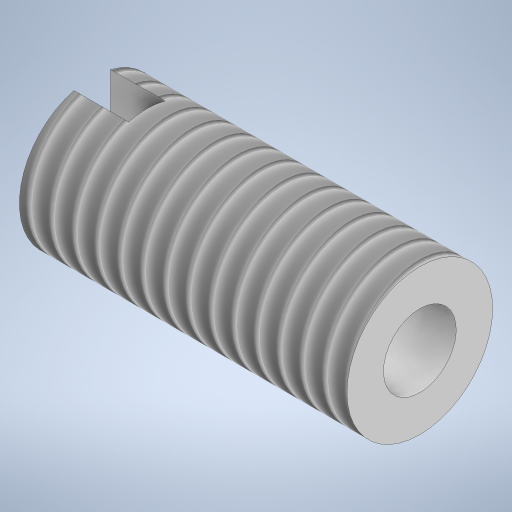
# Autodesk Inventor part: HUDSON-1-89B
Saved by Autodesk Inventor 2024.2 (Build 282272000, 272)
## iProperties
Created: 2024-10-06
Part Number: HUDSON-1-89B
Material: Generic
Document SubType Name: Modeling
Designer: melim
Density: 1 g/cm^3
Appearance: Default
Author: melim
Autodesk Inventor part; units mm, degrees
ref_plane "YZ Plane" through (0, 0, 0) normal (1, 0, 0) x (0, 1, 0)
ref_plane "XY Plane" through (0, 0, 0) normal (0, 0, 1) x (1, 0, 0)
sketch "Sketch1" plane through (0, 0, 0) normal (1, 0, 0) x (0, 1, 0)
  circle A0 centre (0, 0) radius 4
  circle A1 centre (0, 0) radius 2
  dimension "d0" = 8
  dimension "d1" = 4
  constraints: 2 centre point, 2 coincident
  measures "d0" diameter of A0
  measures "d1" diameter of A1
extrude "Extrusion1" add sketch "Sketch1" along normal blind 18
ref_plane "Work Plane1" through (0, 4, 0) normal (0, 1, 0) x (-1, 0, 0)
sketch "Sketch2" plane through (0, 4, 0) normal (0, 1, 0) x (-1, 0, 0)
  line L0 (-18, 4) -> (-18, -4) projected
  line L1 (0, 4) -> (0, -4) projected
  line L2 (1, 1) -> (-3, 1)
  line L3 (-3, 1) -> (-3, -1)
  line L4 (-3, -1) -> (1, -1)
  line L5 (1, -1) -> (1, 1)
  point P0 (0, 0)
  point P1 (-1, -1)
  point P2 (0, 0)
  dimension "d4" = 1
  dimension "d5" = 1
  dimension "d6" = 3
  constraints: 8 end point, 2 midpoint, 2 parallel, 1 horizontal, 1 perpendicular
  measures "d4" horizontal distance of point (-1, -1) point (0, 0)
  measures "d5" distance from line of point (0, 0) L2
  measures "d6" distance from line of L2.end L1
extrude "Extrusion2" cut sketch "Sketch2" against normal through all
thread "Thread1" size "M8x1.25" class "6g" standard "ANSI Metric M Profile" full length
body "Solid1"
